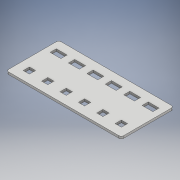
# Autodesk Inventor part: CuvetteRack-250x144
Saved by Autodesk Inventor 2017 (Build 210142000, 142)
## iProperties
Created: 2021-07-06
Part Number: CuvetteRack-250x144
Material: Generic
Document SubType Name: Modeling
Designer: Nikita
Density: 1 g/cm^3
Appearance: Default
Author: Nikita
Autodesk Inventor part; units mm, degrees
ref_plane "YZ Plane" through (0, 0, 0) normal (1, 0, 0) x (0, 1, 0)
ref_plane "XZ Plane" through (0, 0, 0) normal (0, 1, 0) x (-1, 0, 0)
ref_plane "XY Plane" through (0, 0, 0) normal (0, 0, 1) x (1, 0, 0)
sketch "Sketch1" plane through (0, 0, 0) normal (0, 0, 1) x (1, 0, 0)
  line L0 (0.2549, 114.5315) -> (250.2549, 114.5315)
  line L1 (250.2549, 114.5315) -> (250.2549, 0.5315)
  line L2 (250.2549, 0.5315) -> (0.2549, 0.5315)
  line L3 (0.2549, 0.5315) -> (0.2549, 114.5315)
  line L4 (14.3894, 96.0315) -> (37.0049, 96.0315)
  line L5 (37.0049, 96.0315) -> (37.0049, 82.5315)
  line L6 (37.0049, 82.5315) -> (13.5049, 82.5315)
  line L7 (13.5049, 82.5315) -> (13.5049, 96.0315)
  line L8 (18.5049, 32.5315) -> (32.0049, 32.5315)
  line L9 (32.0049, 32.5315) -> (32.0049, 19.0315)
  line L10 (32.0049, 19.0315) -> (18.5049, 19.0315)
  line L11 (18.5049, 19.0315) -> (18.5049, 32.5315)
  line L12 (77.0049, 96.0315) -> (77.0049, 82.5315)
  line L13 (77.0049, 82.5315) -> (53.5049, 82.5315)
  line L14 (53.5049, 82.5315) -> (53.5049, 96.0315)
  line L15 (53.5049, 96.0315) -> (77.0049, 96.0315)
  line L16 (117.0049, 96.0315) -> (117.0049, 82.5315)
  line L17 (117.0049, 82.5315) -> (93.5049, 82.5315)
  line L18 (93.5049, 82.5315) -> (93.5049, 96.0315)
  line L19 (93.5049, 96.0315) -> (117.0049, 96.0315)
  line L20 (157.0049, 96.0315) -> (157.0049, 82.5315)
  line L21 (157.0049, 82.5315) -> (133.5049, 82.5315)
  line L22 (133.5049, 82.5315) -> (133.5049, 96.0315)
  line L23 (133.5049, 96.0315) -> (157.0049, 96.0315)
  line L24 (197.0049, 96.0315) -> (197.0049, 82.5315)
  line L25 (197.0049, 82.5315) -> (173.5049, 82.5315)
  line L26 (173.5049, 82.5315) -> (173.5049, 96.0315)
  line L27 (173.5049, 96.0315) -> (197.0049, 96.0315)
  line L28 (237.0049, 96.0315) -> (237.0049, 82.5315)
  line L29 (237.0049, 82.5315) -> (213.5049, 82.5315)
  line L30 (213.5049, 82.5315) -> (213.5049, 96.0315)
  line L31 (213.5049, 96.0315) -> (237.0049, 96.0315)
  line L32 (72.0049, 32.5315) -> (72.0049, 19.0315)
  line L33 (72.0049, 19.0315) -> (58.5049, 19.0315)
  line L34 (58.5049, 19.0315) -> (58.5049, 32.5315)
  line L35 (58.5049, 32.5315) -> (72.0049, 32.5315)
  line L36 (112.0049, 32.5315) -> (112.0049, 19.0315)
  line L37 (112.0049, 19.0315) -> (98.5049, 19.0315)
  line L38 (98.5049, 19.0315) -> (98.5049, 32.5315)
  line L39 (98.5049, 32.5315) -> (112.0049, 32.5315)
  line L40 (152.0049, 32.5315) -> (152.0049, 19.0315)
  line L41 (152.0049, 19.0315) -> (138.5049, 19.0315)
  line L42 (138.5049, 19.0315) -> (138.5049, 32.5315)
  line L43 (138.5049, 32.5315) -> (152.0049, 32.5315)
  line L44 (192.0049, 32.5315) -> (192.0049, 19.0315)
  line L45 (192.0049, 19.0315) -> (178.5049, 19.0315)
  line L46 (178.5049, 19.0315) -> (178.5049, 32.5315)
  line L47 (178.5049, 32.5315) -> (192.0049, 32.5315)
  line L48 (232.0049, 32.5315) -> (232.0049, 19.0315)
  line L49 (232.0049, 19.0315) -> (218.5049, 19.0315)
  line L50 (218.5049, 19.0315) -> (218.5049, 32.5315)
  line L51 (218.5049, 32.5315) -> (232.0049, 32.5315)
  line L52 (25.2549, 68.2407) -> (25.2549, 48.1897)
  line L53 (34.2286, 57.5315) -> (15.7703, 57.5315)
  line L54 (14.3894, 96.0315) -> (13.5049, 96.0315)
  point P0 (0, 0)
  dimension "d8" = 250
  dimension "d9" = 114
  dimension "d10" = 23.5
  dimension "d11" = 13.5
  dimension "d12" = 13.5
  dimension "d13" = 13.5
  dimension "d14" = 40
  dimension "d15" = 40
  dimension "d16" = 13.25
  dimension "d19" = 50
  constraints: 110 end point, 7 horizontal, 6 parallel, 3 perpendicular, 1 vertical, 84 other
  measures "d8" distance of L2.start L2.end
  measures "d9" distance of L0.end L2.start
  measures "d10" distance of L6.start L6.end
  measures "d11" distance of L4.end L6.start
  measures "d12" distance of L10.start L10.end
  measures "d13" distance of L8.end L10.start
  measures "d14" distance of L7.end L14.end
  measures "d15" distance of L8.end L35.end
  measures "d16" distance between parallel lines of L3 L7
  measures "d19" diameter of L6 L53
extrude "Extrusion1" add sketch "Sketch1" along normal blind 5
fillet "Fillet1" radius 5 4 edges at (250.2549, 114.5315, 2.5) (250.2549, 0.5315, 2.5) (0.2549, 114.5315, 2.5) (0.2549, 0.5315, 2.5)
body "Solid1"
